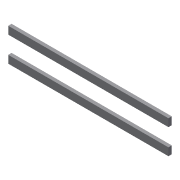
# Autodesk Inventor part: Fan_oulet
Saved by Autodesk Inventor 2017 (Build 210142000, 142)
## iProperties
Created: 2018-04-20
Part Number: Fan_oulet
Material: Generic
Document SubType Name: Modeling
Designer: Kathryn Rosie
Density: 1 g/cm^3
Appearance: Default
Author: Kathryn Rosie
Autodesk Inventor part; units mm, degrees
ref_plane "YZ Plane" through (0, 0, 0) normal (1, 0, 0) x (0, 1, 0)
ref_plane "XZ Plane" through (0, 0, 0) normal (0, 1, 0) x (-1, 0, 0)
ref_plane "XY Plane" through (0, 0, 0) normal (0, 0, 1) x (1, 0, 0)
sketch "Sketch1" plane through (0, 0, 0) normal (0, 0, 1) x (1, 0, 0)
  circle A0 centre (-290, -632) radius 55 projected
  line L0 (22, 0) -> (22, -1544) projected
  line L1 (-1022, -1544) -> (-1022, 0) projected
  line L2 (-290, -632) -> (22, -632) construction
  line L3 (22, -575) -> (-1022, -575)
  line L4 (-1022, -575) -> (-1022, -525)
  line L5 (-1022, -525) -> (22, -525)
  line L6 (22, -525) -> (22, -575)
  line L7 (-290, -632) -> (-290, -492.7476) construction
  line L8 (22, -689) -> (-1022, -689)
  line L9 (-1022, -689) -> (-1022, -739)
  line L10 (-1022, -739) -> (22, -739)
  line L11 (22, -739) -> (22, -689)
  point P0 (0, 0)
  point P1 (-290, -771.2524)
  dimension "d1" = 50
  dimension "d2" = 57
  constraints: 20 end point, 5 symmetric about line, 2 horizontal, 2 parallel, 2 point on line, 1 perpendicular, 1 vertical
  measures "d1" distance between parallel lines of L5 L3
  measures "d2" distance from line of L2.start L3
extrude "Extrusion1" add sketch "Sketch1" along normal blind 22 contours L0 L3 L1 L5 | L0 L10 L1 L8
body "Solid1"
